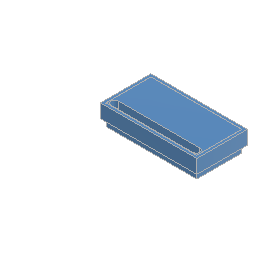
Tweezer-Carrier (Autodesk Fusion 360 design; units mm, degrees)
Autodesk Fusion 360 part; units mm, degrees
sketch "Sketch1" plane through (0, 0, 18.175) normal (0, 0, 1) x (-1, 0, 0)
  line L0 (-2.95, 189.992) -> (-2.95, 140.892)
  line L1 (-2.95, 140.892) -> (-102.05, 140.892)
  line L2 (-102.05, 140.892) -> (-102.05, 189.992)
  line L3 (-102.05, 189.992) -> (-2.95, 189.992)
  line L4 (0, 137.942) -> (0, 192.942)
  line L5 (0, 192.942) -> (-105, 192.942)
  line L6 (-105, 192.942) -> (-105, 137.942)
  line L7 (-105, 137.942) -> (0, 137.942)
  line L8 (-102.05, 140.892) -> (-102.05, 189.992)
  line L9 (-102.05, 189.992) -> (-2.95, 189.992)
  line L10 (-3.05, 140.992) -> (-101.95, 140.992)
  line L11 (-101.95, 140.992) -> (-101.95, 189.892)
  line L12 (-101.95, 189.892) -> (-3.05, 189.892)
  line L13 (-3.05, 189.892) -> (-3.05, 140.992)
  dimension "d173" = 0.1
extrude "Extrude1" add sketch "Sketch1" against normal blind 7.5 contours L10 L11 L12 L13 makes body 1
sketch "Sketch2" plane through (0, 0, 18.175) normal (0, 0, 1) x (-1, 0, 0)
  line L0 (-3.05, 189.892) -> (-101.95, 189.892)
  line L1 (-101.95, 189.892) -> (-101.95, 140.992)
  line L2 (-101.95, 140.992) -> (-3.05, 140.992)
  line L3 (-3.05, 140.992) -> (-3.05, 189.892)
  line L4 (-2.95, 189.992) -> (-2.95, 140.892)
  line L5 (-2.95, 140.892) -> (-102.05, 140.892)
  line L6 (-102.05, 140.892) -> (-102.05, 189.992)
  line L7 (-102.05, 189.992) -> (-2.95, 189.992)
  line L8 (0, 137.942) -> (0, 192.942)
  line L9 (0, 192.942) -> (-105, 192.942)
  line L10 (-105, 192.942) -> (-105, 137.942)
  line L11 (-105, 137.942) -> (0, 137.942)
extrude "Extrude2" add sketch "Sketch2" along normal blind 15 bodies 1 makes body 2 at (70, -137.942, 23.175)
sketch "Sketch3" plane through (0, 0, 33.175) normal (0, 0, 1) x (-1, 0, 0)
  line L0 (-3.05, 140.992) -> (-3.05, 189.892)
  line L1 (-3.05, 189.892) -> (-101.95, 189.892)
  line L2 (-101.95, 189.892) -> (-101.95, 140.992)
  line L3 (-101.95, 140.992) -> (-3.05, 140.992)
  line L4 (-96.875, 181.442) -> (-8.125, 181.442)
  arc A0 (-8.125, 181.442) -> (-8.125, 189.442) centre (-8.125, 185.442) ccw
  line L5 (-8.125, 189.442) -> (-96.875, 189.442)
  arc A1 (-96.875, 189.442) -> (-96.875, 181.442) centre (-96.875, 185.442) ccw
  line L6 (-96.875, 185.442) -> (-8.125, 185.442) construction
  line L7 (-105, 192.942) -> (-105, 137.942)
  line L8 (0, 297.942) -> (0, 0)
  line L9 (0, 192.942) -> (-105, 192.942)
  dimension "d179" = 88.75
  dimension "d180" = 8
  dimension "d181" = 8.125
  dimension "d182" = 8.125
  dimension "d183" = 7.5
  constraint tangent L4 A0
  constraint tangent A0 L5
  constraint parallel L4 L5
  constraint tangent L5 A1
  constraint tangent L4 A1
  constraint parallel L1 L6
  measures "d179" distance of A1.centre A0.centre
  measures "d180" diameter of A0
  measures "d181" distance of A1.centre L7
  measures "d182" distance of A0.centre L8
  measures "d183" distance of A1.centre L9
extrude "Extrude3" cut sketch "Sketch3" against normal blind 8 contours L4 A0 L5 A1 bodies 1
equation "d173 = SmallTolerence * 2"
equation "d174 = -InsertLockDepth"
equation "d176 = TweezerCarrierDepth"
equation "d179 = TweezerCarrierTweezerLength - ( TweezerCarrierTweezerWidth )"
equation "d180 = TweezerCarrierTweezerWidth"
equation "d184 = -TweezerCarrierTweezerWidth"
equation "SmallTolerence = 0.05 mm"
equation "InsertLockDepth = 7.5 mm"
equation "TweezerCarrierTweezerLength = 96.75 mm"
equation "TweezerCarrierTweezerWidth = 8 mm"
equation "TweezerCarrierDepth = 15 mm"
